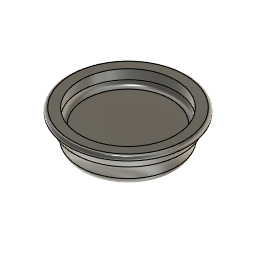
Cahssis Sketch v2 (Autodesk Fusion 360 archive; units mm, degrees)
design "Castor Wheel Holder"
Autodesk Fusion 360 part; units mm, degrees
sketch "Sketch1" plane through (0, 0, 0) normal (0, 0, 1) x (1, 0, 0)
  circle A0 centre (0, 0) radius 17
  circle A1 centre (0, 0) radius 25
  dimension "d1" = 34
  dimension "d2" = 50
  constraint coincident A0.centre A1.centre
  measures "d1" diameter of A0
  measures "d2" diameter of A1
ref_plane "WorkPlane1" through (0, 0, 12) normal (0, 0, 1) x (1, 0, 0)
sketch "Sketch2" plane through (0, 0, 12) normal (0, 0, 1) x (1, 0, 0)
  circle A0 centre (0, 0) radius 32.5
  dimension "d4" = 65
  constraint coincident A0.centre origin
  measures "d4" diameter of A0
loft "Loft1" add profiles "Sketch2", "Sketch1" section 1 section 2
extrude "Extrude1" add sketch "Sketch1" against normal blind 6.5
fillet "Fillet1" radius 1.5 1 edges at (-30.3006, 11.7525, 12)
fillet "Fillet2" radius 20 1 edges at (-23.3082, -9.0404, 0)
fillet "Fillet3" radius 5 1 edges at (-23.3082, 9.0404, -6.5)
sketch "Sketch3" plane through (0, 0, 12) normal (0, 0, 1) x (-1, 0, 0)
  circle A0 centre (0, 0) radius 29.7936
  circle A1 centre (0, 0) radius 25
  dimension "d13" = 50
  constraint coincident A0.centre A1.centre
  measures "d13" diameter of A1
extrude "Extrude2" cut sketch "Sketch3" against normal blind 7.5 contours A1
fillet "Fillet4" radius 2.5 1 edges at (23.3082, -9.0404, 4.5)
